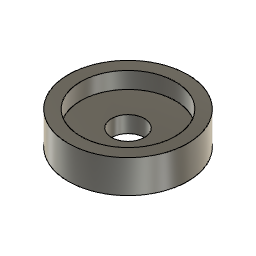
screw+washer (Autodesk Fusion 360 design; units mm, degrees)
Autodesk Fusion 360 part; units mm, degrees
sketch "Sketch1" plane through (0, 0, 0) normal (0, 0, 1) x (1, 0, 0)
  circle A0 centre (0, 0) radius 5.75
  circle A1 centre (0, 0) radius 7.25
  dimension "d1" = 11.5
  dimension "d9" = 1.5
  constraint coincident A0.centre A1.centre
  constraint concentric A0 A1
  measures "d1" diameter of A0
  measures "d9" distance of A0 A1
extrude "Extrude1" add sketch "Sketch1" along normal blind 4
extrude "Extrude2" add sketch "Sketch1" along normal blind 2 contours A0
sketch "Sketch2" plane through (0, 0, 2) normal (0, 0, 1) x (-1, 0, 0)
  circle A0 centre (0, 0) radius 5.75
  circle A1 centre (0, 0) radius 2
  dimension "d6" = 4
  constraint coincident A0.centre A1.centre
  measures "d6" diameter of A1
extrude "Extrude3" cut sketch "Sketch2" against normal blind 5 contours A1
